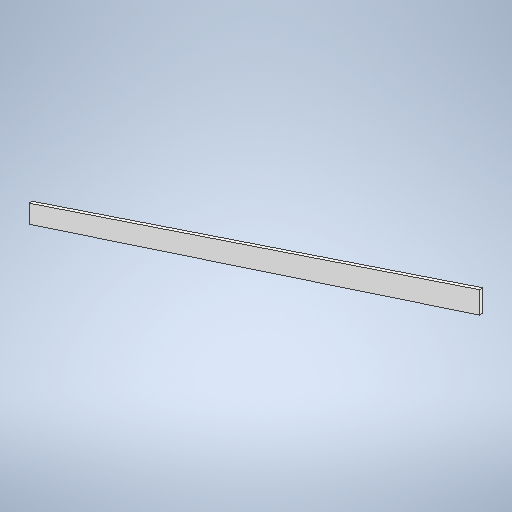
# Autodesk Inventor part: Fascia_For_Side
Saved by Autodesk Inventor 2025.1 (Build 291241020, 241B)
## iProperties
Created: 2024-09-15
Part Number: Fascia_For_Side
Material: Generic
Document SubType Name: Modeling
Designer: Tom
Density: 1 g/cm^3
Appearance: White
Author: Tom
Autodesk Inventor part; units mm, degrees
ref_plane "XZ Plane" through (0, 0, 0) normal (0, 1, 0) x (-1, 0, 0)
ref_plane "XY Plane" through (0, 0, 0) normal (0, 0, 1) x (1, 0, 0)
sketch "Sketch1" plane through (0, 0, 0) normal (0, 0, 1) x (1, 0, 0)
  line L0 (0, 0) -> (3321.2151, 1108.1486)
  line L1 (3321.2151, 1255.4197) -> (-136.6838, 101.6655)
  line L2 (0, 0) -> (-136.6838, 0)
  line L3 (-136.6838, 0) -> (-136.6838, 101.6655)
  line L4 (-136.6838, 101.6655) -> (1593.1098, 678.8242)
  line L5 (3321.2151, 1108.1486) -> (3263.9, 1108.1486)
  line L6 (3321.2151, 1108.1486) -> (3321.2151, 1255.4197)
  line L7 (-88.9, 0) -> (-88.9, 117.6089)
  line L8 (3263.9, 1089.025) -> (3263.9, 1236.2961)
  line L9 (-136.6838, 101.6655) -> (-136.6838, -38.0345)
  line L10 (-136.6838, -38.0345) -> (3321.2151, 1086.4335)
  line L11 (3321.2151, 1086.4335) -> (3321.2151, 1108.1486)
  dimension "d5" = 139.7
  dimension "d17" = 88.9
  dimension "d19" = 3352.8
  dimension "d23" = 57.3151
  dimension "d28" = 47.7837
  dimension "d33" = 1089.025
  dimension "d36" = 139.7
  dimension "d37" = 168.9862
  constraints: 24 end point, 5 point on line, 5 vertical, 2 coincident, 2 collinear, 2 horizontal
  measures "d5" distance between parallel lines of L1 L0
  measures "d17" distance from line of L7 point (0, 0)
  measures "d19" distance between parallel lines of L7 L8
  measures "d23" distance between parallel lines of L6 L8
  measures "d28" distance between parallel lines of L3 L7
  measures "d33" vertical distance of L8.start point (0, 0)
  measures "d36" distance of L1.end L9.end
  measures "d37" distance of L1.start L10.end
extrude "Extrusion2" add sketch "Sketch1" along normal blind 25.4 contours L8 L5 L0 | L0 L11 L10 | L0 L10 L2 L7 L1 L8 | L5 L8 L1 L6 | L10 L9 L2 | L2 L3 L1 L7
ref_plane "Work Plane2" through (-136.6838, -38.0345, 0) normal (0, 1, 0) x (0, 0, 1)
body "Solid2"
